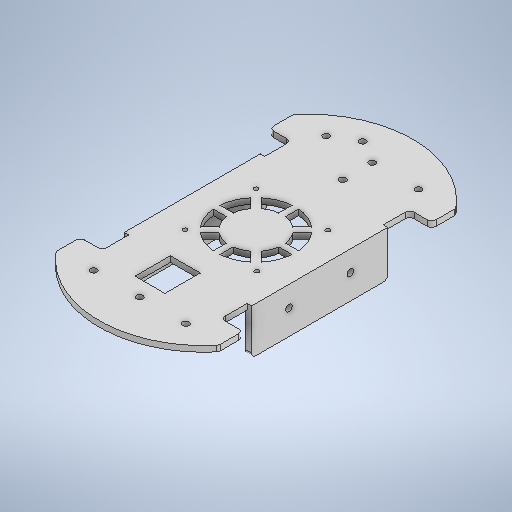
# Autodesk Inventor part: module_part1_fan
Saved by Autodesk Inventor 2025.2 (Build 292293000, 293)
## iProperties
Created: 2025-05-02
Part Number: module_part1_fan
Material: Generic
Document SubType Name: Modeling
Designer: holz
Density: 1 g/cm^3
Appearance: Default
Author: holz
Autodesk Inventor part; units mm, degrees
ref_plane "YZ Plane" through (0, 0, 0) normal (1, 0, 0) x (0, 1, 0)
ref_plane "XZ Plane" through (0, 0, 0) normal (0, 1, 0) x (-1, 0, 0)
ref_plane "XY Plane" through (0, 0, 0) normal (0, 0, 1) x (1, 0, 0)
sketch "Sketch1" plane through (0, 0, 0) normal (0, 1, 0) x (-1, 0, 0)
  line L0 (0, 0) -> (-74, 0)
  line L1 (-74, -86) -> (-74, -86)
  line L2 (-74, -86) -> (0, -86)
  line L3 (0, -86) -> (0, -97)
  line L4 (0, -97) -> (-74, -97)
  line L5 (-74, -97) -> (-74, -86)
  line L6 (-74, 0) -> (0, 0)
  line L7 (0, 0) -> (0, 11)
  line L8 (0, 11) -> (-74, 11)
  line L9 (-74, 11) -> (-74, 0)
  line L10 (-74, 11) -> (0, 11)
  line L11 (0, 11) -> (0, 28.5)
  line L12 (0, 28.5) -> (-74, 28.5)
  line L13 (-74, 28.5) -> (-74, 11)
  line L14 (-74, -97) -> (0, -97)
  line L15 (0, -97) -> (0, -114.5)
  line L16 (0, -114.5) -> (-74, -114.5)
  line L17 (-74, -114.5) -> (-74, -97)
  arc A0 (0, 11) -> (-74, 11) centre (-37, -19.3643) ccw
  arc A1 (-74, -97) -> (0, -97) centre (-37, -66.6357) ccw
  line L18 (-37, 0) -> (-65, 0)
  line L19 (-69, -86) -> (-39, -86)
  line L20 (-37, 0) -> (-5, 0)
  line L21 (-9, -86) -> (-39, -86)
  line L22 (-9, -86) -> (-10, -86)
  line L23 (-10, -86) -> (-10, 0)
  line L24 (-10, 0) -> (-8, 0)
  line L25 (-69, -86) -> (-66, -86)
  line L26 (-66, 0) -> (-65, 0)
  line L27 (0, 11) -> (-74, 11)
  line L28 (-74, 11) -> (-74, -49.7286)
  line L29 (-74, -49.7286) -> (0, -49.7286)
  line L30 (0, -49.7286) -> (0, 11)
  line L31 (-37, -49.7286) -> (-37, -97)
  line L32 (-37, -49.7286) -> (-37, 0)
  line L33 (-37, -97) -> (-10, -97)
  line L34 (-9, 0) -> (-37, 0)
  line L35 (-37, 0) -> (-37, -97)
  line L36 (-37, 0) -> (-64, 0)
  line L37 (-64, 0) -> (-64, -86)
  line L38 (-64, -86) -> (-37, -86)
  line L39 (-37, -86) -> (-37, 0)
  point P0 (-10, 0)
  dimension "d1" = 86
  dimension "d2" = 11
  dimension "d3" = 11
  dimension "d4" = 17.5
  dimension "d5" = 17.5
  dimension "d11" = 74
  dimension "d12" = 74
  dimension "d15" = 27
  dimension "d16" = 27
  constraints: 80 end point, 18 parallel, 12 horizontal, 8 point on line, 7 perpendicular, 6 point on circle, 5 midpoint, 2 centre point, 2 tangent, 1 collinear
  measures "d1" distance of L1.start L0.end
  measures "d2" distance of L2.end L3.end
  measures "d3" distance of L7.end L6.end
  measures "d4" distance of L11.end L10.end
  measures "d5" distance of L14.end L15.end
  measures "d11" distance of L7.end L8.end
  measures "d12" distance of L3.end L4.end
  measures "d15" distance of L23.end L36.start
  measures "d16" distance of L36.end L34.end
extrude "Extrusion1" add sketch "Sketch1" against normal blind 2.6 contours L0 L9 L8 L7 | L8 A0 | L29 L32 L0 L23 | L23 L2 L31 L29 | L2 L3 L4 L31 | L31 L2 L37 L29 | L29 L37 L0 L32 | L31 L4 L5 L2 | L4 A1
fillet "Face Fillet1" radius 2 1 edges at (74, -1.3, -86)
fillet "Face Fillet2" radius 2 1 edges at (64, -1.3, -86)
fillet "Face Fillet3" radius 2 1 edges at (74, -1.3, 11)
fillet "Face Fillet4" radius 2 1 edges at (0, -1.3, -86)
fillet "Face Fillet5" radius 2 1 edges at (0, -1.3, 11)
fillet "Face Fillet6" radius 2 1 edges at (0, -1.3, 0)
fillet "Face Fillet7" radius 2 1 edges at (0, -1.3, -97)
fillet "Face Fillet8" radius 2 1 edges at (74, -1.3, -97)
fillet "Face Fillet9" radius 2 1 edges at (74, -1.3, 0)
sketch "Sketch2" plane through (3.0029, 0, 0.2026) normal (0, 1, 0) x (1, 0, 0)
  line L0 (7.3045, 43.1826) -> (61.3045, 43.1826)
  circle A0 centre (33.9975, 43.1826) radius 12
  circle A1 centre (33.9975, 43.1826) radius 18
  line L1 (59.2562, 43.1826) -> (12.239, 43.1826)
  line L2 (12.239, 43.1826) -> (12.239, 41.6826)
  line L3 (12.239, 41.6826) -> (59.2562, 41.6826)
  line L4 (12.239, 43.1826) -> (59.2562, 43.1826)
  line L5 (59.2562, 44.6826) -> (12.239, 44.6826)
  line L6 (12.239, 44.6826) -> (12.239, 43.1826)
  line L7 (33.9975, 67.2692) -> (35.4975, 67.2692)
  line L8 (35.4975, 67.2692) -> (35.4975, 19.3724)
  line L9 (35.4975, 19.3724) -> (33.9975, 19.3724)
  line L10 (33.9975, 19.3724) -> (33.9975, 67.2692)
  line L11 (33.9975, 19.3724) -> (32.4975, 19.3724)
  line L12 (32.4975, 19.3724) -> (32.4975, 67.2692)
  line L13 (32.4975, 67.2692) -> (33.9975, 67.2692)
  line L14 (33.9975, 67.2692) -> (33.9975, 19.3724)
  line L15 (26.0457, 51.1345) -> (41.8772, 35.303)
  line L16 (24.2706, 33.4557) -> (40.1021, 49.2872)
  line L17 (36.0724, 41.1077) -> (47.8222, 29.358)
  line L18 (47.8222, 29.358) -> (18.8436, 58.3365)
  line L19 (48.5938, 57.7789) -> (20.866, 30.0511)
  line L20 (48.5938, 57.7789) -> (20.866, 30.0511)
  line L21 (20.866, 30.0511) -> (19.716, 31.2011)
  line L22 (19.716, 31.2011) -> (47.4438, 58.9289)
  line L23 (48.5938, 57.7789) -> (20.866, 30.0511)
  line L24 (20.866, 30.0511) -> (22.016, 28.9011)
  line L25 (22.016, 28.9011) -> (49.7438, 56.6289)
  line L26 (18.8436, 58.3365) -> (47.8222, 29.358)
  line L27 (46.6722, 28.208) -> (17.6936, 57.1865)
  line L28 (17.6936, 57.1865) -> (18.8436, 58.3365)
  line L29 (18.8436, 58.3365) -> (47.8222, 29.358)
  line L30 (48.9722, 30.508) -> (19.9936, 59.4865)
  line L31 (19.9936, 59.4865) -> (18.8436, 58.3365)
  line L32 (6.9971, 0.2026) -> (6.9971, 86.2026) projected
  line L33 (60.9971, 84.2026) -> (60.9971, 0.2026) projected
  line L34 (6.9971, 86.2026) -> (60.9971, 86.2026)
  line L35 (60.9971, 86.2026) -> (60.9971, 0.2026)
  line L36 (60.9971, 0.2026) -> (6.9971, 0.2026)
  line L37 (6.9971, 0.2026) -> (6.9971, 86.2026)
  line L38 (6.9971, 86.2026) -> (60.9971, 86.2026)
  line L39 (60.9971, 86.2026) -> (60.9971, 63.2691)
  line L40 (6.9971, 63.2691) -> (6.9971, 86.2026)
  line L41 (-1.0029, 0.2026) -> (6.9971, 0.2026) projected
  line L42 (6.9971, 0.2026) -> (60.9971, 0.2026)
  line L43 (60.9971, 0.2026) -> (60.9971, 27.2691)
  line L44 (61.558, 25.1826) -> (7.558, 25.1826)
  line L45 (6.9971, 27.2691) -> (6.9971, 0.2026)
  line L46 (6.9971, 25.2021) -> (6.9971, 27.2691)
  line L47 (47.4438, 58.9289) -> (49.7438, 56.6289)
  line L48 (59.2562, 44.6826) -> (59.2562, 41.6826)
  line L49 (46.6722, 28.208) -> (48.9722, 30.508)
  line L50 (6.9971, 0.2026) -> (64.4943, 0.2026)
  line L51 (6.9971, 25.2021) -> (6.9971, 0.2026)
  line L52 (6.9971, 86.2026) -> (71.9441, 86.2026)
  line L53 (6.6901, 61.1826) -> (6.9971, 86.2026)
  line L54 (6.6901, 61.1826) -> (15.6901, 61.1826)
  line L55 (15.6901, 61.1826) -> (15.6901, 5.8279)
  line L56 (15.6901, 5.8279) -> (6.6901, 5.8279)
  line L57 (6.6901, 5.8279) -> (6.6901, 61.1826)
  line L58 (60.9971, 65.7254) -> (51.9975, 65.7254)
  line L59 (51.9975, 65.7254) -> (51.9975, 14.7661)
  line L60 (51.9975, 14.7661) -> (60.9971, 14.7661)
  line L61 (60.9971, 14.7661) -> (60.9971, 65.7254)
  point P0 (0, 0)
  point P1 (22.4717, 57.0085)
  point P2 (26.7405, 52.7396)
  point P3 (32.4975, 55.0885)
  point P4 (32.4975, 61.12)
  point P5 (24.4405, 50.4396)
  point P6 (20.1717, 54.7085)
  point P7 (16.0601, 44.6826)
  point P8 (22.0917, 44.6826)
  point P9 (20.1717, 31.6568)
  point P10 (24.4405, 35.9257)
  point P11 (22.0917, 41.6826)
  point P12 (16.0601, 41.6826)
  point P13 (26.7405, 33.6257)
  point P14 (22.4717, 29.3568)
  point P15 (32.4975, 25.2453)
  point P16 (32.4975, 31.2768)
  point P17 (45.5234, 29.3568)
  point P18 (41.2545, 33.6256)
  point P19 (35.4975, 31.2768)
  point P20 (35.4975, 25.2453)
  point P21 (43.5545, 35.9256)
  point P22 (47.8234, 31.6568)
  point P23 (51.9349, 41.6826)
  point P24 (45.9034, 41.6826)
  point P25 (47.8234, 54.7085)
  point P26 (43.5545, 50.4396)
  point P27 (45.9034, 44.6826)
  point P28 (51.9349, 44.6826)
  point P29 (41.2545, 52.7396)
  point P30 (45.5234, 57.0085)
  point P31 (35.4975, 61.12)
  point P32 (35.4975, 55.0885)
  dimension "d46" = 9
  dimension "d47" = 8.9995
  constraints: 118 end point, 19 parallel, 12 horizontal, 12 perpendicular, 5 point on line, 2 centre point, 2 collinear, 2 vertical, 1 coincident
  measures "d46" distance of L55.end L56.end
  measures "d47" distance of L59.end L60.end
extrude "Extrusion2" cut sketch "Sketch2" along normal mid plane 40 contours A0 L25 A1 L5 | L3 A1 L30 A0 | A0 L8 A1 L22 | L27 A1 L8 A0 | A1 L25 A0 L12 | L5 A1 L27 A0 | A0 L22 A1 L3 | A0 L30 A1 L12
fillet "Face Fillet10" radius 2 1 edges at (10, -1.3, -86)
fillet "Face Fillet11" radius 2 1 edges at (10, -1.3, 0)
fillet "Face Fillet12" radius 2 1 edges at (64, -1.3, 0)
sketch "Sketch3" plane through (0, 0, 0) normal (0, 1, 0) x (1, 0, 0)
  arc A0 (64, 2) -> (66, 0) centre (66, 2) ccw projected
  line L0 (10, 2) -> (66, 2)
  line L1 (66, 2) -> (66, 0)
  line L2 (66, 0) -> (10, 0)
  line L3 (66, 2) -> (8, 2)
  line L4 (8, 2) -> (8, 0)
  line L5 (8, 0) -> (66, 0)
  line L6 (66, 0) -> (66, 2)
  line L7 (64, 84) -> (64, 2) projected
  line L8 (10, 0) -> (64, 0)
  line L9 (64, 0) -> (64, 12)
  line L10 (64, 12) -> (10, 12)
  line L11 (10, 12) -> (10, 0)
  line L12 (10, 2) -> (10, 84) projected
  line L13 (10, 20.306) -> (29, 20.306)
  line L14 (29, 20.306) -> (29, 0)
  line L15 (29, 0) -> (10, 0)
  line L16 (10, 0) -> (10, 20.306)
  line L17 (64, 0) -> (40, 0)
  line L18 (40, 0) -> (40, 20.6777)
  line L19 (40, 20.6777) -> (64, 20.6777)
  line L20 (64, 20.6777) -> (64, 0)
  line L21 (40, 0) -> (29, 0)
  line L22 (29, 0) -> (29, 13.8728)
  line L23 (40, 13.5728) -> (40, 0)
  line L24 (29, 0) -> (41.0276, 0)
  line L25 (41.0276, 0) -> (41.0276, -1.3)
  line L26 (41.0276, -1.3) -> (29, -1.3)
  line L27 (29, -1.3) -> (29, 0)
  line L28 (40, 13.3) -> (41.3, 13.3)
  line L29 (41.3, 13.3) -> (41.3, -1.3)
  line L30 (41.3, -1.3) -> (40, -1.3)
  line L31 (40, -1.3) -> (40, 13.3)
  line L32 (29, 16.2654) -> (27.7, 16.2654)
  line L33 (27.7, 16.2654) -> (27.7, -1.3)
  line L34 (27.7, -1.3) -> (29, -1.3)
  line L35 (29, -1.3) -> (29, 16.2654)
  line L36 (27.7, 12) -> (41.3, 12)
  line L37 (41.3, 12) -> (41.3, 13.3)
  line L38 (41.3, 13.3) -> (27.7, 13.3)
  line L39 (27.7, 13.3) -> (27.7, 12)
  line L40 (28.35, -1.3) -> (28.35, 0)
  point P0 (0, 0)
  point P1 (41.0276, -1.3)
  dimension "d51" = 12
  dimension "d52" = 19
  dimension "d53" = 24
  dimension "d54" = 1.3
  dimension "d55" = 1.3
  dimension "d56" = 1.3
  dimension "d57" = 1.3
  constraints: 78 end point, 18 parallel, 11 perpendicular, 11 point on line, 10 horizontal, 1 midpoint
  measures "d51" distance of L10.end L2.end
  measures "d52" distance of L13.start L13.end
  measures "d53" distance of L18.end L19.end
  measures "d54" distance of L36.end L28.end
  measures "d55" distance of L40.end L40.start
  measures "d56" distance of L33.end L26.end
  measures "d57" distance of L28.end L28.start
extrude "Extrusion3" cut sketch "Sketch3" along normal mid plane 40 contours L29 L2 L18 L0 | L0 L18 L10 L29 | L18 L2 L14 L0 | L0 L14 L10 L18 | L10 L18 L28 L29 | L29 L30 L25 L2 | L14 L2 L33 L0 | L0 L33 L10 L14 | L31 L26 L27 L2 | L2 L25 L26 L31 | L10 L14 L38 L18 | L10 L33 L38 L14 | L27 L34 L40 L2 | L2 L40 L34 L33
sketch "Sketch8" plane through (64, -2.6, -84) normal (1, 0, 0) x (0, 0, -1)
  line L0 (-82, 0) -> (0, 0) projected
  line L1 (-82, 0) -> (0, 0)
  line L2 (0, 0) -> (0, 18)
  line L3 (0, 18) -> (-82, 18)
  line L4 (-82, 18) -> (-82, 0)
  line L5 (-82, 2.6) -> (0, 2.6) projected
  line L6 (-41, 0) -> (-41, 18)
  line L7 (-41, 18) -> (-72, 18)
  line L8 (-72, 18) -> (-72, 0)
  line L9 (-72, 0) -> (-41, 0)
  line L10 (-41, 0) -> (-41, 18)
  line L11 (-41, 18) -> (-10, 18)
  line L12 (-10, 18) -> (-10, 0)
  line L13 (-10, 0) -> (-41, 0)
  line L14 (-41, 0) -> (-41, 18)
  line L15 (-10, 18) -> (-72, 18)
  line L16 (-72, 18) -> (-72, -18)
  line L17 (-72, -18) -> (-10, -18)
  line L18 (-10, -18) -> (-10, 18)
  line L19 (-41, 18) -> (-41, -27.3873)
  line L20 (-72, 2.6) -> (-10, 2.6)
  line L21 (-10, 2.6) -> (-10, -1.4102)
  line L22 (-10, -1.4102) -> (-72, -1.4102)
  line L23 (-72, -1.4102) -> (-72, 2.6)
  point P0 (-84, 2.6)
  point P1 (-72, 0)
  point P2 (-10, 0)
  point P3 (-10, 18)
  point P4 (-10, 0)
  point P5 (-10, 2.6)
  point P6 (-72, 2.6)
  point P7 (-72, 0)
  dimension "d87" = 18
  dimension "d88" = 82
  dimension "d89" = 31
  dimension "d90" = 31
  dimension "d125" = 18
  constraints: 44 end point, 11 parallel, 6 point on line, 5 perpendicular, 4 horizontal, 2 midpoint
  measures "d87" distance of L1.end L2.end
  measures "d88" distance of L2.end L3.end
  measures "d89" distance of L6.end L11.end
  measures "d90" distance of L7.end L6.end
  measures "d125" distance of L17.end L12.end
sketch "Sketch9" plane through (10, -2.6, -84) normal (-1, 0, 0) x (0, 0, 1)
  line L0 (0, 2.6) -> (0, 0) projected
  line L1 (0, 0) -> (72.0022, 0)
  line L2 (72.0022, 0) -> (72.0022, 18)
  line L3 (72.0022, 18) -> (0, 18)
  line L4 (0, 18) -> (0, 0)
  line L5 (82, 2.6) -> (0, 2.6) projected
  line L6 (41, 2.6) -> (10, 2.6)
  line L7 (10, 2.6) -> (10, 18)
  line L8 (10, 18) -> (41, 18)
  line L9 (41, 18) -> (41, 2.6)
  line L10 (72.0022, 18) -> (10, 18)
  line L11 (10, 18) -> (10, 0)
  line L12 (10, 0) -> (72.0022, 0)
  line L13 (72.0022, 0) -> (72.0022, 18)
  line L14 (72.0022, 18) -> (10, 18)
  line L15 (10, 18) -> (10, -18)
  line L16 (10, -18) -> (72.0022, -18)
  line L17 (72.0022, -18) -> (72.0022, 18)
  line L18 (72.0022, 0) -> (10, 0)
  line L19 (10, 0) -> (10, -18)
  line L20 (10, -18) -> (72.0022, -18)
  line L21 (72.0022, -18) -> (72.0022, 0)
  line L22 (72.0022, 0) -> (10, 0)
  line L23 (10, 0) -> (10, 2.6)
  line L24 (10, 2.6) -> (72.0022, 2.6)
  line L25 (72.0022, 2.6) -> (72.0022, 0)
  line L26 (41, 18) -> (41.0011, -18)
  point P0 (84, 2.6)
  point P1 (10, 18)
  point P2 (10, 2.6)
  point P3 (72.0022, 2.6)
  point P4 (10, 2.6)
  point P5 (10, 0)
  dimension "d1" = 86
  dimension "d2" = 11
  dimension "d3" = 11
  dimension "d4" = 17.5
  dimension "d5" = 17.5
  dimension "d11" = 74
  dimension "d12" = 74
  dimension "d15" = 27
  dimension "d16" = 27
  dimension "d91" = 31
  dimension "d92" = 18
  dimension "d126" = 20.6
  constraints: 50 end point, 12 parallel, 6 horizontal, 6 perpendicular, 2 midpoint, 1 point on line
  measures "d91" distance of L7.end L8.end
  measures "d92" distance of L10.end L11.end
  measures "d126" distance of L15.end L6.end
sketch "Sketch4" plane through (0, 0, 0) normal (0, 1, 0) x (1, 0, 0)
  line L0 (41.3, -1.3) -> (27.7, -1.3) projected
  line L1 (41.3, -1.3) -> (27.7, -1.3)
  line L2 (27.7, -1.3) -> (27.7, -2.8)
  line L3 (27.7, -2.8) -> (41.3, -2.8)
  line L4 (41.3, -2.8) -> (41.3, -1.3)
  point P0 (0, 0)
  dimension "d60" = 1.5
  constraints: 8 end point, 2 parallel, 1 horizontal, 1 perpendicular
  measures "d60" distance of L1.end L2.end
extrude "Extrusion4" cut sketch "Sketch4" along normal mid plane 40
sketch "Sketch5" plane through (0, 0, 0) normal (0, 1, 0) x (1, 0, 0)
  arc A0 (10, 84) -> (8, 86) centre (8, 84) ccw projected
  line L0 (64, 2) -> (64, 84) projected
  line L1 (10, 84) -> (64, 84)
  line L2 (64, 84) -> (64, 71.4558)
  line L3 (64, 71.4558) -> (10, 71.4558)
  line L4 (10, 71.4558) -> (10, 84)
  line L5 (37, 84) -> (37, 60.4451)
  line L6 (26.2602, 84) -> (40.4168, 84)
  line L7 (40.4168, 84) -> (40.4168, 82.5)
  line L8 (40.4168, 82.5) -> (26.2602, 82.5)
  line L9 (26.2602, 82.5) -> (26.2602, 84)
  circle A1 centre (37, 82.5) radius 1.5
  line L10 (8, 86) -> (2, 86) projected
  line L11 (2, 86) -> (74.2134, 86)
  line L12 (70.1915, 96) -> (-2.0219, 96)
  line L13 (70.1915, 96) -> (-4.0219, 96)
  line L14 (-4.0219, 96) -> (-4.0219, 86)
  line L15 (-4.0219, 86) -> (70.1915, 86)
  line L16 (74, 96.2758) -> (74, 88) projected
  line L17 (74, 88) -> (74, 85.5591)
  line L18 (74, 85.5591) -> (74, 96)
  line L19 (37, 84) -> (37, 116.0596)
  line L20 (37, 100.0298) -> (16, 100.0298)
  line L21 (16, 100.0298) -> (16, 86)
  line L22 (16, 86) -> (37, 86)
  line L23 (37, 86) -> (37, 100.0298)
  line L24 (37, 105.7284) -> (58, 105.7284)
  line L25 (58, 105.7284) -> (58, 86)
  line L26 (58, 86) -> (37, 86)
  line L27 (37, 86) -> (37, 105.7284)
  line L28 (16, 100.0298) -> (0, 100.0298)
  line L29 (0, 100.0298) -> (0, 86)
  line L30 (0, 86) -> (16, 86)
  line L31 (16, 86) -> (16, 100.0298)
  line L32 (58, 100.874) -> (74, 100.874)
  line L33 (74, 100.874) -> (74, 86)
  line L34 (74, 86) -> (58, 86)
  line L35 (58, 86) -> (58, 100.874)
  line L36 (10.4417, 86) -> (6.2096, 86)
  line L37 (6.2096, 86) -> (6.2096, 96)
  line L38 (6.2096, 96) -> (10.4417, 96)
  line L39 (10.4417, 96) -> (10.4417, 86)
  circle A2 centre (16, 96) radius 1.45
  circle A3 centre (37, 96) radius 1.45
  circle A4 centre (58, 96) radius 1.45
  line L40 (16, 96) -> (58, 96)
  line L41 (58, 96) -> (58, -18.2327)
  line L42 (58, -18.2327) -> (16, -18.2327)
  line L43 (16, -18.2327) -> (16, 96)
  line L44 (37, 100.0298) -> (37, -18.2327)
  line L45 (71.1847, 0) -> (5, 0)
  line L46 (5, 0) -> (5, -10)
  line L47 (5, -10) -> (71.1847, -10)
  line L48 (71.1847, -10) -> (71.1847, 0)
  circle A5 centre (58, -10) radius 1.5
  circle A6 centre (37, -10) radius 1.5
  circle A7 centre (16, -10) radius 1.5
  point P0 (0, 0)
  dimension "d63" = 1.5
  dimension "d64" = 3
  dimension "d65" = 21
  dimension "d66" = 21
  dimension "d67" = 10
  dimension "d68" = 2.9
  dimension "d69" = 2.9
  dimension "d70" = 2.9
  dimension "d71" = 10
  dimension "d72" = 3
  dimension "d73" = 3
  dimension "d74" = 3
  constraints: 92 end point, 27 point on line, 20 parallel, 11 horizontal, 10 perpendicular, 7 centre point, 3 midpoint, 3 vertical, 1 collinear
  measures "d63" distance of L7.end L6.end
  measures "d64" diameter of A1
  measures "d65" distance of L20.start L20.end
  measures "d66" distance of L24.start L24.end
  measures "d67" distance of L38.end L36.start
  measures "d68" diameter of A3
  measures "d69" diameter of A4
  measures "d70" diameter of A2
  measures "d71" distance of L45.end L46.end
  measures "d72" diameter of A7
  measures "d73" diameter of A6
  measures "d74" diameter of A5
sketch "Sketch6" plane through (0, 0, 0) normal (0, 1, 0) x (1, 0, 0)
  line L0 (63.6416, 43.8178) -> (45.6416, 43.8178)
  line L1 (45.6416, 43.8178) -> (45.6416, 91.2338)
  line L2 (45.6416, 91.2338) -> (63.6416, 91.2338)
  line L3 (63.6416, 91.2338) -> (63.6416, 43.8178)
  line L4 (45.6416, 86.1637) -> (41.2249, 86.1637)
  line L5 (41.2249, 86.1637) -> (41.2249, 103.2333)
  line L6 (41.2249, 103.2333) -> (45.6416, 103.2333)
  line L7 (45.6416, 103.2333) -> (45.6416, 86.1637)
  line L8 (8.4008, 86.1637) -> (26.4008, 86.1637)
  line L9 (26.4008, 86.1637) -> (26.4008, 102.1637)
  line L10 (26.4008, 102.1637) -> (8.4008, 102.1637)
  line L11 (8.4008, 102.1637) -> (8.4008, 86.1637)
  circle A0 centre (26.4008, 102.1637) radius 1.5
  point P0 (0, 0)
  dimension "d75" = 18
  dimension "d76" = 18
  dimension "d77" = 3
  dimension "d124" = 16
  constraints: 24 end point, 6 parallel, 4 horizontal, 3 perpendicular, 1 centre point, 1 coincident, 1 point on line, 1 vertical
  measures "d75" distance of L1.end L2.end
  measures "d76" distance of L9.end L10.end
  measures "d77" diameter of A0
  measures "d124" distance of L8.end L9.end
sketch "Sketch7" plane through (0, 0, 0) normal (0, 1, 0) x (1, 0, 0)
  line L0 (74.426, 0) -> (58.0542, 0)
  line L1 (58.0542, 0) -> (58.0542, 26.3227)
  line L2 (74.426, 86.149) -> (4.426, 86.149)
  line L3 (4.426, 86.149) -> (4.426, 59.249)
  line L4 (4.426, 59.249) -> (74.426, 59.249)
  line L5 (74.426, 59.249) -> (74.426, 86.149)
  line L6 (72, 0) -> (66, 0) projected
  line L7 (69, 0) -> (-3.2352, 0)
  line L8 (-3.2352, 0) -> (-3.2352, 26.9)
  line L9 (-3.2352, 26.9) -> (69, 26.9)
  line L10 (69, 26.9) -> (69, 0)
  line L11 (10.2495, 8.087) -> (20.7495, 8.087)
  line L12 (20.7495, 8.087) -> (20.7495, 77.4568)
  line L13 (20.7495, 77.4568) -> (10.2495, 77.4568)
  line L14 (10.2495, 77.4568) -> (10.2495, 8.087)
  line L15 (64, 84) -> (64, 2) projected
  line L16 (64, 3.1555) -> (53.5, 3.1555)
  line L17 (53.5, 3.1555) -> (53.5, 80.3103)
  line L18 (53.5, 80.3103) -> (64, 80.3103)
  line L19 (64, 80.3103) -> (64, 3.1555)
  circle A0 centre (53.5, 26.9) radius 1
  circle A1 centre (53.5, 59.249) radius 1
  circle A2 centre (20.7495, 26.9) radius 1
  circle A3 centre (20.7495, 59.249) radius 1
  point P0 (0, 0)
  dimension "d78" = 26.9
  dimension "d79" = 70
  dimension "d80" = 26.9
  dimension "d81" = 10.5
  dimension "d82" = 10.5
  dimension "d83" = 2
  dimension "d84" = 2
  dimension "d85" = 2
  dimension "d86" = 2
  constraints: 36 end point, 9 point on line, 8 parallel, 6 horizontal, 5 perpendicular, 4 centre point, 1 midpoint, 1 vertical
  measures "d78" distance of L2.end L3.end
  measures "d79" distance of L3.end L4.end
  measures "d80" distance of L7.end L8.end
  measures "d81" distance of L11.start L11.end
  measures "d82" distance of L16.start L16.end
  measures "d83" diameter of A3
  measures "d84" diameter of A2
  measures "d85" diameter of A0
  measures "d86" diameter of A1
extrude "Extrusion11" cut sketch "Sketch7" against normal blind 10 contours A0 L17 L9 | L9 L17 A0 | L17 A0 L9 | L9 A0 L17 | A1 L17 L4 | L4 L17 A1 | A1 L4 L17 | L4 A1 L17 | A2 L12 L9 | L9 L12 A2 | A2 L12 L9 | L9 L12 A2 | A3 L12 L4 | L4 L12 A3 | A3 L12 L4 | L4 L12 A3
extrude "Extrusion12" cut sketch "Sketch5" against normal blind 10 contours A1 L8 L5 | L5 L8 A1 | A2 L12 L21 | L21 L12 A2 | A2 L21 L12 | L8 A1 L5 | L5 A1 L8 | A7 L47 L43 | L43 L47 A7 | A3 L12 L19 | L19 L12 A3 | L21 A2 L12 | L47 A7 L43 | L43 A7 L47 | A6 L47 L44 | L44 L47 A6 | A4 L12 L25 | L25 L12 A4 | L19 A3 L12 | L12 A3 L19 | A5 L47 L41 | L41 L47 A5 | L47 L44 A6 | L47 A6 L44 | L25 A4 L12 | L12 A4 L25 | L47 A5 L41 | L41 A5 L47
extrude "Extrusion13" cut sketch "Sketch6" against normal blind 10 contours A0 L10 L9 | L9 L10 A0
extrude "Extrusion14" add sketch "Sketch9" along normal blind 2 and the other way blind 1 contours L5 L26 L1 L11 | L1 L26 L16 L15 | L5 L2 L1 L26 | L1 L17 L16 L26
extrude "Extrusion15" add sketch "Sketch8" along normal blind 2 and the other way blind 1 contours L8 L5 L6 L0 | L0 L19 L22 L16 | L6 L5 L12 L0 | L0 L18 L22 L19 | L22 L19 L17 L16 | L22 L18 L17 L19
fillet "Face Fillet17" radius 2 1 edges at (64.5, -20.6, -74)
fillet "Face Fillet18" radius 2 1 edges at (9.5, -20.6, -74)
fillet "Face Fillet19" radius 2 1 edges at (9.5, -20.6, -11.9978)
fillet "Face Fillet20" radius 2 1 edges at (64.5, -20.6, -12)
sketch "Sketch15" plane through (66, -2.6, -84) normal (1, 0, 0) x (0, 0, -1)
  line L0 (-12, -18) -> (-70, -18) projected
  line L1 (-41, -18) -> (-41, 2.6)
  line L2 (-10, 2.6) -> (-72, 2.6) projected
  line L3 (-41, -18) -> (-55, -18)
  line L4 (-55, -18) -> (-55, 4.5909)
  line L5 (-55, 4.5909) -> (-41, 4.5909)
  line L6 (-41, 4.5909) -> (-41, -18)
  line L7 (-41, -18) -> (-27, -18)
  line L8 (-27, -18) -> (-27, 5.0171)
  line L9 (-27, 5.0171) -> (-41, 5.0171)
  line L10 (-41, 5.0171) -> (-41, -18)
  line L11 (-21.635, 2.5955) -> (-60.0211, 2.5955)
  line L12 (-60.0211, 2.5955) -> (-60.0211, -6.7045)
  line L13 (-60.0211, -6.7045) -> (-21.635, -6.7045)
  line L14 (-21.635, -6.7045) -> (-21.635, 2.5955)
  circle A0 centre (-27, -6.7045) radius 1.5
  circle A1 centre (-55, -6.7045) radius 1.5
  point P0 (-84, 2.6)
  dimension "d139" = 14
  dimension "d140" = 14
  dimension "d141" = 9.3
  dimension "d142" = 3
  dimension "d143" = 3
  constraints: 26 end point, 6 parallel, 3 horizontal, 3 midpoint, 3 perpendicular, 3 point on line, 2 centre point
  measures "d139" distance of L4.end L5.end
  measures "d140" distance of L8.end L9.end
  measures "d141" distance of L13.end L11.start
  measures "d142" diameter of A0
  measures "d143" diameter of A1
sketch "Sketch16" plane through (8, -2.6, -84) normal (-1, 0, 0) x (0, 0, 1)
  circle A0 centre (27, -6.7045) radius 1.5
  circle A1 centre (55, -6.7045) radius 1.5
  point P0 (84, 2.6)
  dimension "d144" = 3
  dimension "d145" = 3
  constraints: 2 centre point
  measures "d144" diameter of A0
  measures "d145" diameter of A1
extrude "Extrusion16" cut sketch "Sketch16" along normal blind 40 and the other way blind 5
extrude "Extrusion17" cut sketch "Sketch15" along normal blind 40 and the other way blind 20 contours A0 L13 L8 | L8 L13 A0 | L13 A0 L8 | L8 A0 L13 | A1 L13 L4 | L4 L13 A1 | L13 L4 A1 | L13 A1 L4
body "Solid1"
